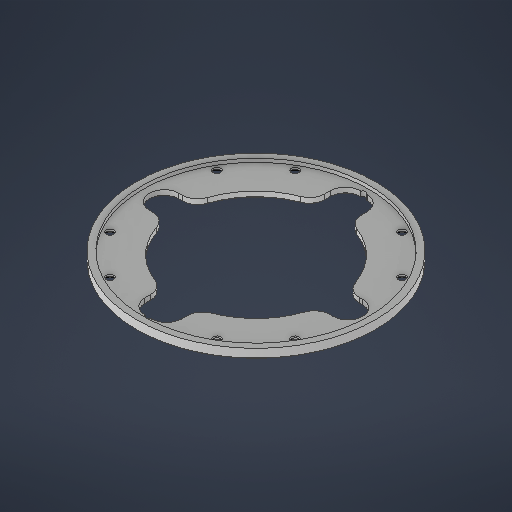
# Autodesk Inventor part: Clamp Ring
Saved by Autodesk Inventor 2025 (Build 290162000, 162)
## iProperties
Created: 2024-08-23
Part Number: Clamp Ring
Material: Generic
Document SubType Name: Modeling
Designer: mayhe
Density: 1 g/cm^3
Appearance: Default
Author: mayhe
Autodesk Inventor part; units mm, degrees
ref_plane "YZ Plane" through (0, 0, 0) normal (1, 0, 0) x (0, 1, 0)
ref_plane "XZ Plane" through (0, 0, 0) normal (0, 1, 0) x (-1, 0, 0)
ref_plane "XY Plane" through (0, 0, 0) normal (0, 0, 1) x (1, 0, 0)
sketch "Sketch1" plane through (0, 0, 0) normal (0, 1, 0) x (-1, 0, 0)
  circle A0 centre (0, 0) radius 85
  circle A1 centre (0, 0) radius 80.5
  line L0 (75.9132, 0) -> (75.9132, 0)
  line L1 (-75.9132, 0) -> (-75.9132, 0)
  line L2 (-75.9132, 6.869) -> (75.9132, -6.869) construction
  line L3 (75.9132, 14.131) -> (-75.9132, -14.131) construction
  line L4 (2.5, 76.5) -> (-2.5, 76.5)
  line L5 (-2.5, -76.5) -> (2.5, -76.5)
  line L6 (13, 76.5) -> (-13, -76.5) construction
  line L7 (-13, 76.5) -> (13, -76.5) construction
  arc A2 (13, 66) -> (2.5, 76.5) centre (2.5, 66) ccw
  arc A3 (-2.5, 76.5) -> (-13, 66) centre (-2.5, 66) ccw
  arc A4 (-65.4132, 10.5) -> (-75.9132, 0) centre (-65.4132, 0) ccw
  arc A5 (-75.9132, 0) -> (-65.4132, -10.5) centre (-65.4132, 0) ccw
  arc A6 (75.9132, 0) -> (65.4132, 10.5) centre (65.4132, 0) ccw
  arc A7 (65.4132, -10.5) -> (75.9132, 0) centre (65.4132, 0) ccw
  arc A8 (2.5, -76.5) -> (13, -66) centre (2.5, -66) ccw
  arc A9 (-13, -66) -> (-2.5, -76.5) centre (-2.5, -66) ccw
  line L8 (13, -66) -> (13, -62.0181)
  line L9 (13, 62.0181) -> (13, 66)
  line L10 (62.9285, 10.5) -> (65.4132, 10.5)
  line L11 (-65.4132, 10.5) -> (-62.9285, 10.5)
  line L12 (-13, 66) -> (-13, 62.0181)
  line L13 (-13, -62.0181) -> (-13, -66)
  line L14 (65.4132, -10.5) -> (62.9285, -10.5)
  line L15 (-62.9285, -10.5) -> (-65.4132, -10.5)
  arc A10 (20.0301, -51.7595) -> (52.5193, -17.9436) centre (0, 0) ccw
  arc A11 (52.5193, 17.9436) -> (20.0301, 51.7595) centre (0, 0) ccw
  arc A12 (-20.0301, 51.7595) -> (-52.5193, 17.9436) centre (0, 0) ccw
  arc A13 (-52.5193, -17.9436) -> (-20.0301, -51.7595) centre (0, 0) ccw
  arc A14 (-62.9285, 10.5) -> (-52.5193, 17.9436) centre (-62.9285, 21.5) ccw
  arc A15 (-52.5193, -17.9436) -> (-62.9285, -10.5) centre (-62.9285, -21.5) ccw
  arc A16 (-13, -62.0181) -> (-20.0301, -51.7595) centre (-24, -62.0181) ccw
  arc A17 (20.0301, -51.7595) -> (13, -62.0181) centre (24, -62.0181) ccw
  arc A18 (62.9285, -10.5) -> (52.5193, -17.9436) centre (62.9285, -21.5) ccw
  arc A19 (52.5193, 17.9436) -> (62.9285, 10.5) centre (62.9285, 21.5) ccw
  arc A20 (13, 62.0181) -> (20.0301, 51.7595) centre (24, 62.0181) ccw
  arc A21 (-20.0301, 51.7595) -> (-13, 62.0181) centre (-24, 62.0181) ccw
  point P0 (-13, -53.956)
  point P1 (13, -53.956)
  point P2 (13, 53.956)
  point P3 (-13, 53.956)
  point P4 (54.4977, -10.5)
  point P5 (54.4977, 10.5)
  point P6 (-54.4977, 10.5)
  point P7 (-54.4977, -10.5)
  point P8 (75.9132, 0)
  point P9 (-75.9132, 0)
  dimension "d0" = 170
  dimension "d1" = 161
  dimension "d3" = 152
  dimension "d4" = 21
  dimension "d5" = 26
  dimension "d6" = 153
  dimension "d7" = 10.5
  dimension "d8" = 10.5
  dimension "d9" = 11
  constraints: 48 point on circle, 40 tangent, 32 end point, 22 centre point, 16 point on line, 13 equal radius, 10 parallel, 4 midpoint, 4 perpendicular, 3 coincident, 3 horizontal
  measures "d0" diameter of A0
  measures "d1" diameter of A1
  measures "d3" distance of L2.end L3.end
  measures "d4" distance of L3.start L2.end
  measures "d5" distance of L7.end L6.end
  measures "d6" distance of L6.end L7.start
  measures "d7" radius of A2
  measures "d8" radius of A3
  measures "d9" radius of A14
extrude "Extrusion1" add sketch "Sketch1" along normal blind 6.5 contours A0
extrude "Extrusion2" add sketch "Sketch1" along normal blind 4 contours A1
sketch "Sketch2" plane through (0, 0, 0) normal (0, -1, 0) x (1, 0, 0)
  circle A0 centre (0, 0) radius 76
  circle A1 centre (0, 76) radius 1
  circle A2 centre (0, -76) radius 1
  circle A3 centre (0, -76) radius 2.75
  circle A4 centre (38, -65.8179) radius 2.75
  circle A5 centre (65.8179, -38) radius 2.75
  circle A6 centre (76, 0) radius 2.75
  circle A7 centre (65.8179, 38) radius 2.75
  circle A8 centre (38, 65.8179) radius 2.75
  circle A9 centre (0, 76) radius 2.75
  circle A10 centre (-38, 65.8179) radius 2.75
  circle A11 centre (-65.8179, 38) radius 2.75
  circle A12 centre (-76, 0) radius 2.75
  circle A13 centre (-65.8179, -38) radius 2.75
  circle A14 centre (-38, -65.8179) radius 2.75
  dimension "d14" = 152
  dimension "d15" = 2
  dimension "d16" = 2
  dimension "d17" = 5.5
  dimension "d20" = 360
  constraints: 15 centre point, 2 coincident, 2 point on circle, 25 other
  measures "d14" diameter of A0
  measures "d15" diameter of A1
  measures "d16" diameter of A2
  measures "d17" diameter of A3
extrude "Extrusion3" cut sketch "Sketch2" against normal blind 4 contours A7 A0 | A0 A7 | A5 A0 | A0 A5 | A8 A0 | A0 A8 | A4 A0 | A0 A4 | A10 A0 | A0 A10 | A14 A0 | A0 A14 | A11 A0 | A0 A11 | A13 A0 | A0 A13
hole "Hole1" at (0, 0, 76) at (0, 0, -76) direction (0, 1, 0) diameter 4 depth 8.8
chamfer "Chamfer2" distance 0.5 angle 45 33 edges at (9.9246, 0, -73.4246) (13, 0, -64.0091) (14.9262, 0, -55.8) (40.0216, 0, -38.4515) (56.5301, 0, -12.5524) (64.1709, 0, -10.5) (75.9132, 0, 0) (64.1709, 0, 10.5) (56.5301, 0, 12.5524) (40.0216, 0, 38.4515) (14.9262, 0, 55.8) (13, 0, 64.0091) (9.9246, 0, 73.4246) (2.2182, 0, 76.5) (2.2182, 0, -76.5) (0, 0, -78) (-9.9246, 0, -73.4246) (-2.2182, 0, -76.5) (-13, 0, -64.0091) (-14.9262, 0, -55.8) (-40.0216, 0, -38.4515) (-56.5301, 0, -12.5524) (-64.1709, 0, -10.5) (-75.9132, 0, 0) (-64.1709, 0, 10.5) (-56.5301, 0, 12.5524) (-40.0216, 0, 38.4515) (-14.9262, 0, 55.8) (-13, 0, 64.0091) (-9.9246, 0, 73.4246) (-2.2182, 0, 76.5) (0, 0, 78) (85, 0, 0)
hole "Hole2" at (-38, 0, -65.8179) at (38, 0, -65.8179) at (65.8179, 0, -38) at (65.8179, 0, 38) at (38, 0, 65.8179) at (-38, 0, 65.8179) at (-65.8179, 0, 38) at (-65.8179, 0, -38) direction (0, 1, 0) diameter 4.134 depth 14.2 countersink diameter 11.2 countersink angle 90 thread size "M5x0.8" class "6H" standard "ISO Metric profile"
body "Solid1"
